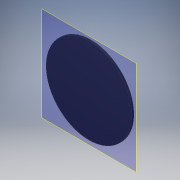
# Autodesk Inventor part: capot inférieur
Saved by Autodesk Inventor 2018 (Build 220112000, 112)
## iProperties
Created: 2017-10-08
Part Number: capot inférieur
Material: Iron, Cast
Document SubType Name: Modeling
Designer: liamg
Density: 7.15 g/cm^3
Appearance: Iron Gray
Author: liamg
Autodesk Inventor part; units mm, degrees
ref_plane "YZ Plane" through (0, 0, 0) normal (1, 0, 0) x (0, 1, 0)
ref_plane "XZ Plane" through (0, 0, 0) normal (0, 1, 0) x (-1, 0, 0)
ref_plane "XY Plane" through (0, 0, 0) normal (0, 0, 1) x (1, 0, 0)
ref_plane "Work Plane1" through (-1.0629, 12.8024, 9.5903) normal (0, 0, -1) x (-1, 0, 0)
sketch "Sketch1" plane through (-1.0629, 12.8024, 9.5903) normal (0, 0, -1) x (-1, 0, 0)
  circle A0 centre (0, 0) radius 17.93 projected
  point P0 (-1.0629, -12.8024)
extrude "Extrusion1" add sketch "Sketch1" along normal blind 0.8
body "Solid1"
